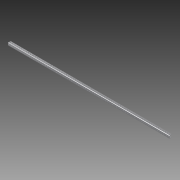
# Autodesk Inventor part: DBK_C-Channel_72
Saved by Autodesk Inventor 2014 (Build 180170000, 170)
## iProperties
Category: Drive Base Kit
Company: Autodesk Inc.
Created: 2012-12-27
Part Number: DBK_C-Channel_72
Material: Aluminum 6061
Document SubType Name: Modeling
Designer: Autodesk Inc.
Density: 1 g/cm^3
Catalog Web Link: www.andymark.com
Vendor: AndyMark Inc.
Appearance: Aluminum - Flat
Author: Autodesk Inc.
Autodesk Inventor part; units mm, degrees
ref_plane "YZ Plane" through (0, 0, 0) normal (1, 0, 0) x (0, 1, 0)
ref_plane "XZ Plane" through (0, 0, 0) normal (0, 1, 0) x (-1, 0, 0)
ref_plane "XY Plane" through (0, 0, 0) normal (0, 0, 1) x (1, 0, 0)
sketch "Sketch1" plane through (0, 0, 0) normal (0, 0, 1) x (1, 0, 0)
  line L0 (6.35, 28.575) -> (25.4, 28.575)
  line L1 (6.35, 31.75) -> (25.4, 31.75)
  line L2 (25.4, 0) -> (6.35, 0)
  arc A0 (0, 6.35) -> (6.35, 0) centre (6.35, 6.35) ccw
  line L3 (0, 6.35) -> (0, 25.4)
  arc A1 (6.35, 31.75) -> (0, 25.4) centre (6.35, 25.4) ccw
  line L4 (6.35, 31.75) -> (25.4, 31.75)
  line L5 (25.4, 28.575) -> (6.35, 28.575)
  arc A2 (6.35, 28.575) -> (3.175, 25.4) centre (6.35, 25.4) ccw
  line L6 (3.175, 25.4) -> (3.175, 6.35)
  arc A3 (3.175, 6.35) -> (6.35, 3.175) centre (6.35, 6.35) ccw
  line L7 (6.35, 3.175) -> (25.4, 3.175)
  line L8 (28.575, 3.175) -> (28.575, 0)
  line L9 (25.4, 31.75) -> (28.575, 31.75)
  line L10 (28.575, 28.575) -> (25.4, 28.575)
  line L11 (28.575, 31.75) -> (28.575, 28.575)
  line L12 (28.575, 0) -> (25.4, 0)
  line L13 (28.575, 3.175) -> (28.575, 0)
  line L14 (25.4, 3.175) -> (28.575, 3.175)
  point P0 (0, 0)
  constraints: 30 end point, 8 point on circle, 4 centre point
extrude "Extrusion1" add sketch "Sketch1" against normal blind 1828.8
chamfer "Chamfer1" distance 3.175 angle 45 4 edges at (28.575, 30.1625, 0) (28.575, 1.5875, 0) (28.575, 30.1625, -1828.8) (28.575, 1.5875, -1828.8)
sketch "Sketch2" plane through (6.35, 31.75, 0) normal (0, 1, 0) x (1, 0, 0)
  line L0 (19.05, 0) -> (0, 0) projected
  line L1 (22.225, 3.175) -> (22.225, 1825.625) projected
  point P0 (-6.35, 0)
  point P1 (9.525, 12.7)
  dimension "d5" = 12.7
  dimension "d6" = 12.7
  measures "d5" distance from line of point (9.525, 12.7) L0
  measures "d6" distance from line of point (9.525, 12.7) L1
hole "Hole1" at (15.875, 31.75, -12.7) direction (0, -1, 0) diameter 6.7056 end through all
pattern_linear "Rectangular Pattern1" count 72 spacing 25.4 along (0, 0, -1) of "Hole1"
hole "Hole2" at (0, 15.875, -12.7) direction (1, 0, 0) diameter 6.35 end through all
pattern_linear "Rectangular Pattern2" count 72 spacing 25.4 along (0, 0, -1) of "Hole2"
body "Solid1"
